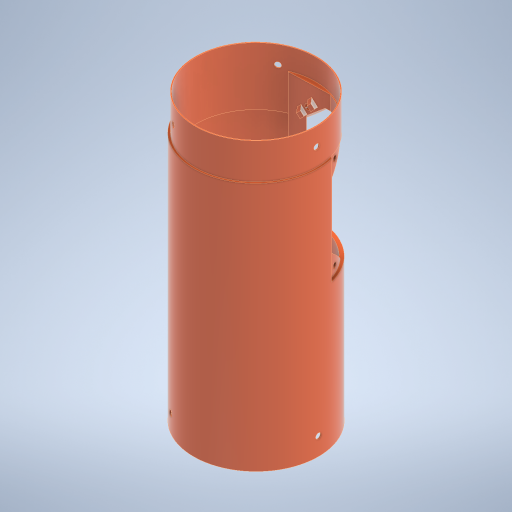
# Autodesk Inventor part: Lower skin
Saved by Autodesk Inventor 2024 (Build 280153000, 153)
## iProperties
Created: 2023-12-30
Part Number: Lower skin
Material: Plastic, Opaque White
Document SubType Name: Modeling
Designer: Jamie
Density: 0.952 g/cm^3
Appearance: Smooth - Light Orange
Author: Jamie
Autodesk Inventor part; units mm, degrees
ref_plane "XY Plane" through (0, 0, 0) normal (0, 0, 1) x (1, 0, 0)
sketch "Sketch1" plane through (0, 0, 0) normal (0, 1, 0) x (-1, 0, 0)
  circle A0 centre (0, 0) radius 35
  circle A1 centre (0, 0) radius 34.5
  dimension "d0" = 70
  dimension "d1" = 69
  constraints: 2 centre point, 2 coincident
  measures "d0" diameter of A0
  measures "d1" diameter of A1
extrude "Extrusion1" add sketch "Sketch1" along normal blind 140
ref_plane "Work Plane2" through (35, 0, 0) normal (1, 0, 0) x (0, 1, 0)
sketch "Sketch4" plane through (35, 0, 0) normal (1, 0, 0) x (0, 1, 0)
  line L0 (140, -35) -> (140, 35) projected
  point P0 (0, 0)
  point P1 (10, 0)
  dimension "d48" = 10
  measures "d48" distance of point (0, 0) point (10, 0)
hole "Hole2" at (35, 10, 0) direction (-1, 0, 0) diameter 3 depth 8 tip angle 118
sketch "Sketch5" plane through (0, 140, 0) normal (0, 1, 0) x (1, 0, 0)
  circle A0 centre (0, 0) radius 34
  circle A1 centre (0, 0) radius 33.5
  dimension "d44" = 68
  dimension "d45" = 67
  constraints: 2 centre point, 2 coincident
  measures "d44" diameter of A0
  measures "d45" diameter of A1
extrude "Extrusion3" add sketch "Sketch5" along normal blind 20
sketch "Sketch6" plane through (0, 140, 0) normal (0, -1, 0) x (1, 0, 0)
  circle A0 centre (0, 0) radius 33.5
  circle A1 centre (0, 0) radius 34.5 projected
  circle A2 centre (0, 0) radius 35
  constraints: 2 centre point, 2 coincident
extrude "Extrusion4" add sketch "Sketch6" along normal blind 12.5 contours A1
ref_plane "Work Plane4" through (34, 0, 0) normal (1, 0, 0) x (0, 1, 0)
sketch "Sketch8" plane through (34, 0, 0) normal (1, 0, 0) x (0, 1, 0)
  line L0 (160, -34) -> (160, 34) projected
  line L1 (150, 0) -> (50.9315, 0)
  line L2 (140, -35) -> (140, 35) projected
  line L3 (130, 15) -> (85, 15)
  line L4 (85, 15) -> (85, -15)
  line L5 (85, -15) -> (130, -15)
  line L6 (130, -15) -> (130, 15)
  point P0 (0, 0)
  point P1 (109.4746, 0)
  dimension "d61" = 10
  dimension "d74" = 15
  dimension "d75" = 10
  dimension "d76" = 15
  dimension "d77" = 55
  constraints: 10 end point, 3 horizontal, 2 parallel, 1 perpendicular
  measures "d61" distance from line of L0 L1.start
  measures "d74" distance from line of L1 L3.start
  measures "d75" distance from line of L2 L3.start
  measures "d76" distance from line of L1 L4.end
  measures "d77" distance from line of L2 L4.end
hole "Hole4" at (34, 150, 0) direction (-1, 0, 0) diameter 3 depth 8 tip angle 118
pattern_circular "Circular Pattern2" count 3 over 360 about axis through (0, 0, 0) along (0, 1, 0) of "Hole2", "Hole4"
sketch "Sketch27" plane through (0, 160, 0) normal (0, 1, 0) x (1, 0, 0)
  circle A0 centre (0, 0) radius 33.5 projected
  line L0 (-15.7198, 29.5827) -> (33.4973, -0.4287) construction
  line L1 (8.8889, 14.5769) -> (24.1701, 39.6371) construction
  circle A1 centre (0, 0) radius 35 construction
  point P0 (18.2219, 29.8825)
  dimension "d174" = 57.6455
  dimension "d175" = 28.823
  dimension "d176" = 0
  constraints: 4 end point, 2 point on circle, 1 perpendicular, 1 point on line, 2 other
  measures "d174" distance of L0.start L0.end
  measures "d175" distance of L0.start L1.start
  measures "d176" distance from line of L1 point (18.222, 29.882)
ref_plane "Work Plane12" through (18.2219, 160, -29.8825) normal (0.5206264, 0, -0.8537846) x (0, 1, 0)
sketch "Sketch28" plane through (18.2219, 160, -29.8825) normal (0.5206264, 0, -0.8537846) x (0, 1, 0)
  line L0 (-20, -35) -> (-20, 35) projected
  line L1 (-17.8725, 0) -> (-86.782, 0) construction
  line L2 (-20, 30) -> (-80, 30)
  line L3 (-80, 30) -> (-80, -30)
  line L4 (-80, -30) -> (-20, -30)
  line L5 (-20, -30) -> (-20, 30)
  point P0 (-160, 0)
  point P1 (-20, -30)
  dimension "d177" = 0
  dimension "d178" = 60
  dimension "d179" = 30
  dimension "d180" = 30
  constraints: 10 end point, 3 horizontal, 2 parallel, 1 perpendicular
  measures "d177" distance from line of L0 L2.start
  measures "d178" distance from line of L0 L3.end
  measures "d179" distance from line of L2.start L1
  measures "d180" distance from line of L3.end L1
extrude "Extrusion8" cut sketch "Sketch28" against normal blind 10
ref_plane "Work Plane18" through (0, 140, 0) normal (0, 1, 0) x (1, 0, 0)
ref_plane "Work Plane20" through (0, 80, 0) normal (0, 1, 0) x (1, 0, 0)
ref_plane "Work Plane23" through (25.5107, 0, -41.8354) normal (-0.8537846, 0, -0.5206264) x (0, 1, 0)
ref_plane "Work Plane21" through (-7.8977, 0, -34.0973) normal (-0.2256487, 0, -0.9742087) x (0, -1, 0)
ref_plane "Work Plane22" through (33.929, 0, -8.5919) normal (0.9694008, 0, -0.2454835) x (0, 1, 0)
ref_plane "Work Plane30" through (0, 110, 0) normal (0, 1, 0) x (1, 0, 0)
sketch "Sketch58" plane through (0, 127.5, 0) normal (0, -1, 0) x (1, 0, 0)
  line L0 (0, 0) -> (-6.1673, -33.7438) construction
  arc A0 (-6.023, -32.9541) -> (32.0543, -9.7351) centre (0, 0) ccw construction
  line L1 (0, 0) -> (32.9079, -9.9944) construction
  line L2 (0, 0) -> (33.3779, -2.8579) construction
  circle A1 centre (0, 0) radius 33.5 construction
  line L3 (0, 0) -> (-12.7429, -30.9817) construction
  arc A2 (32.0543, -9.7351) -> (33.3779, -2.8579) centre (0, 0) ccw
  arc A3 (-12.7429, -30.9817) -> (-6.023, -32.9541) centre (0, 0) ccw
  line L4 (33.3779, -2.8579) -> (34.3742, -2.9432)
  circle A4 centre (0, 0) radius 34.5 projected
  line L5 (-12.7429, -30.9817) -> (-13.1233, -31.9066)
  line L6 (32.0543, -9.7351) -> (33.3094, -8.9698)
  line L7 (33.929, -8.5919) -> (32.6898, -9.3476) projected
  line L8 (-7.2831, -33.7225) -> (-6.023, -32.9541) projected
  line L9 (-7.2831, -33.7225) -> (-6.023, -32.9541)
  point P0 (9.3407, -32.1714)
  point P1 (24.3235, -23.0351)
  point P2 (-7.228, -33.6889)
  point P3 (33.3144, -8.9667)
  dimension "d496" = 12
  dimension "d498" = 12
  dimension "d501" = 33.5
  dimension "d504" = 0
  constraints: 16 end point, 7 point on circle, 2 centre point, 2 line through centre, 2 point on line, 1 coincident, 1 collinear, 1 midpoint
  measures "d496" angle of L2 L1
  measures "d498" angle of L3 L0
  measures "d501" radius of A2
  measures "d504" distance of A3.end L8.end
extrude "Extrusion19" add sketch "Sketch58" along normal blind 47.5 contours A2 L4 A4 L7 L6 | L5 A3 L8 A4
sketch "Sketch59" plane through (0, 80, 0) normal (0, -1, 0) x (1, 0, 0)
  arc A0 (33.3779, -2.8579) -> (-12.7429, -30.9817) centre (0, 0) ccw projected
  line L0 (33.3779, -2.8579) -> (34.3742, -2.9432) projected
  arc A1 (-12.7429, -30.9817) -> (33.3779, -2.8579) centre (0, 0) ccw
  line L1 (33.3779, -2.8579) -> (34.3742, -2.9432)
  line L2 (-12.7429, -30.9817) -> (-13.1211, -31.9075)
  circle A2 centre (0, 0) radius 34.5 projected
  line L3 (-12.7429, -30.9817) -> (-13.1233, -31.9066) projected
  point P0 (32.0543, -9.7351)
  point P1 (-6.023, -32.9541)
  constraints: 4 end point, 3 point on circle, 1 centre point, 1 coincident, 1 collinear, 1 line through centre
extrude "Extrusion20" add sketch "Sketch59" along normal blind 8 contours L0 A2 L2 A1
sketch "Sketch60" plane through (0, 72, 0) normal (0, -1, 0) x (1, 0, 0)
  arc A0 (-12.7429, -30.9817) -> (33.3779, -2.8579) centre (0, 0) ccw projected
  arc A1 (-12.7429, -30.9817) -> (33.3779, -2.8579) centre (0, 0) ccw
  line L0 (-13.1211, -31.9075) -> (-12.7429, -30.9817)
  line L1 (33.3779, -2.8579) -> (34.3742, -2.9432)
  arc A2 (-12.5527, -30.5193) -> (32.8797, -2.8153) centre (0, 0) ccw
  line L2 (-12.5527, -30.5193) -> (-12.7429, -30.9817)
  line L3 (32.8797, -2.8153) -> (33.3779, -2.8579)
  circle A3 centre (0, 0) radius 34.5 projected
  line L4 (-12.5527, -30.5193) -> (10.4338, -31.3071)
  line L5 (32.8797, -2.8153) -> (23.0546, -23.6111)
  point P0 (12.4473, -30.5625)
  dimension "d505" = 33
  dimension "d519" = 23
  dimension "d520" = 23
  constraints: 12 end point, 8 point on circle, 2 centre point, 2 line through centre, 1 coincident, 1 concentric
  measures "d505" radius of A2
  measures "d519" distance of L2.start L4.end
  measures "d520" distance of L3.start L5.end
extrude "Extrusion21" add sketch "Sketch60" against normal blind 76 contours L2 A2 L3 A0 | L4 A2 | A2 L5
sketch "Sketch61" plane through (18.2219, 160, -29.8825) normal (0.5206264, 0, -0.8537846) x (0, 1, 0)
  line L0 (-80, -22.2991) -> (-20, -22.2991) projected
  line L1 (-32.5, -22.2991) -> (-67.5, -22.2991)
  line L2 (-20, 22.2991) -> (-80, 22.2991) projected
  line L3 (-32.5, 22.2991) -> (-67.5, 22.2991)
  line L4 (-32.5, 22.2991) -> (-20, 9.7991)
  line L5 (-20, -23.0434) -> (-20, 23.0434) projected
  line L6 (-20, -34) -> (-20, 34) projected
  line L7 (-20, -9.7991) -> (-32.5, -22.2991)
  line L8 (-67.5, -22.2991) -> (-80, -9.7991)
  line L9 (-80, -9.7991) -> (-80, 9.7991)
  line L10 (-80, -22.2991) -> (-80, 22.2991) projected
  line L11 (-67.5, 22.2991) -> (-80, 9.7991)
  point P0 (-160, 0)
  dimension "d508" = 45
  dimension "d509" = 45
  dimension "d510" = 45
  dimension "d511" = 45
  dimension "d512" = 12.5
  dimension "d513" = 12.5
  dimension "d514" = 12.5
  dimension "d515" = 12.5
  constraints: 14 end point, 7 point on line, 1 vertical
  measures "d508" angle of L11 L10
  measures "d509" angle of L8 L0
  measures "d510" angle of L7 L0
  measures "d511" angle of L5 L4
  measures "d512" distance of L1.start L0.end
  measures "d513" distance of L4.end L2.start
  measures "d514" distance of L2.end L9.end
  measures "d515" distance of L8.end L0.start
extrude "Extrusion22" cut sketch "Sketch61" against normal blind 10 contours L8 L9 L11 L2 L4 L5 L7 L0
sketch "Sketch62" plane through (32.8797, 72, -2.8153) normal (-0.9041677, 0, 0.4271776) x (0.4271776, 0, 0.9041677)
  line L0 (-9.9685, 59.5208) -> (-9.9685, 16.4792) projected
  line L1 (-23, 8) -> (-35.3498, 8) projected
  line L2 (-35.3498, 68) -> (-23, 68) projected
  line L3 (-6.6093, 20.5) -> (-6.6093, 8) projected
  line L4 (-6.6093, 68) -> (-6.6093, 55.5) projected
  point P0 (-11.5, -72)
  point P1 (-10.6093, 12)
  point P2 (-10.6093, 64)
  dimension "d522" = 4
  dimension "d523" = 4
  dimension "d527" = 4
  dimension "d528" = 4
  measures "d522" distance from line of L1 point (-10.609, 12)
  measures "d523" distance from line of L2 point (-10.609, 64)
  measures "d527" distance from line of L3 point (-10.609, 12)
  measures "d528" distance from line of L4 point (-10.609, 64)
hole "Hole25" at (28.3476, 84, -12.4078) at (28.3476, 136, -12.4078) direction (0.9041677, 0, -0.4271776) diameter 3.1 end through all
sketch "Sketch63" plane through (-12.5527, 72, -30.5193) normal (0.0342518, 0, 0.9994132) x (0.9994132, 0, -0.0342518)
  line L0 (23, 68) -> (35.3498, 68) projected
  line L1 (6.6093, 55.5) -> (6.6093, 68) projected
  line L2 (35.3498, 8) -> (23, 8) projected
  line L3 (6.6093, 8) -> (6.6093, 20.5) projected
  point P0 (11.5, -72)
  point P1 (10.6093, 64)
  point P2 (10.6093, 12)
  dimension "d536" = 4
  dimension "d537" = 4
  dimension "d538" = 4
  dimension "d539" = 4
  measures "d536" distance from line of point (10.609, 64) L0
  measures "d537" distance from line of L1 point (10.609, 64)
  measures "d538" distance from line of L2 point (10.609, 12)
  measures "d539" distance from line of L3 point (10.609, 12)
hole "Hole26" at (-1.9496, 136, -30.8827) at (-1.9496, 84, -30.8827) direction (-0.0342518, 0, -0.9994132) diameter 3.1 end through all
sketch "Sketch64" plane through (-12.5527, 72, -30.5193) normal (0.0342518, 0, 0.9994132) x (0.9994132, 0, -0.0342518)
  circle A0 centre (10.6093, 64) radius 2.75 construction
  circle A1 centre (10.6093, 64) radius 1.55 construction
  line L0 (10.7599, 67.668) -> (14.1471, 64.4154)
  line L1 (10.7599, 67.668) -> (12.7938, 69.7862)
  line L2 (12.7938, 69.7862) -> (16.181, 66.5336)
  line L3 (16.181, 66.5336) -> (14.1471, 64.4154)
  circle A2 centre (10.6093, 12) radius 1.55 construction
  line L4 (6.6093, 20.5) -> (9.9685, 16.4792) projected
  point P0 (11.5, -72)
  dimension "d547" = 5.5
  constraints: 8 end point, 2 parallel, 1 centre point, 1 concentric, 1 tangent
  measures "d547" diameter of A0
extrude "Extrusion23" add sketch "Sketch64" along normal blind 2
pattern_circular "Circular Pattern10" count 2 over 360 about axis through (-8.3941, 136, -218.9217) along (0.0342518, 0, 0.9994132) of "Extrusion23"
ref_plane "Work Plane31" through (0, 110, 0) normal (0, 1, 0) x (-1, 0, 0)
mirror "Mirror22" about plane through (0, 110, 0) normal (0, 1, 0) of "Extrusion23", "Circular Pattern10"
sketch "Sketch65" plane through (32.8797, 72, -2.8153) normal (-0.9041677, 0, 0.4271776) x (0.4271776, 0, 0.9041677)
  circle A0 centre (-10.6093, 64) radius 2.75 construction
  circle A1 centre (-10.6093, 64) radius 1.55 construction
  line L0 (-11.2514, 66.9231) -> (-14.9156, 64.2973)
  line L1 (-11.2514, 66.9231) -> (-12.1282, 70.5375)
  line L2 (-12.1282, 70.5375) -> (-15.7924, 67.9117)
  line L3 (-15.7924, 67.9117) -> (-14.9156, 64.2973)
  point P0 (-11.5, -72)
  dimension "d555" = 5.5
  constraints: 8 end point, 2 parallel, 1 centre point, 1 concentric, 1 tangent
  measures "d555" diameter of A0
extrude "Extrusion24" add sketch "Sketch65" along normal blind 2
pattern_circular "Circular Pattern11" count 2 over 360 about axis through (198.4662, 136, -92.7811) along (-0.9041677, 0, 0.4271776) of "Extrusion24"
mirror "Mirror23" about plane through (0, 110, 0) normal (0, 1, 0) of "Extrusion24", "Circular Pattern11"
chamfer "Chamfer25" distance 2 angle 45 1 edges at (25.1078, 141.2246, -14.5834) measured on face at (25.5599, 141.2246, -14.797)
chamfer "Chamfer26" distance 2 angle 45 1 edges at (28.5661, 133.8955, -7.2635) measured on face at (29.0182, 133.8955, -7.4771)
chamfer "Chamfer27" distance 2 angle 45 1 edges at (-0.7143, 140.7271, -28.9239) measured on face at (-0.7314, 140.7271, -29.4236)
chamfer "Chamfer28" distance 2 angle 45 1 edges at (-6.4332, 134.5255, -28.7279) measured on face at (-6.4503, 134.5255, -29.2276)
chamfer "Chamfer29" distance 2 angle 45 1 edges at (-5.757, 88.1599, -28.7511) measured on face at (-5.7741, 88.1599, -29.2508)
chamfer "Chamfer30" distance 2 angle 45 1 edges at (2.671, 82.5255, -29.0399) measured on face at (2.6538, 82.5255, -29.5396)
chamfer "Chamfer31" distance 2 angle 45 1 edges at (27.9708, 89.2246, -8.5236) measured on face at (28.4229, 89.2246, -8.7372)
chamfer "Chamfer32" distance 2 angle 45 1 edges at (24.5125, 81.8955, -15.8435) measured on face at (24.9646, 81.8955, -16.0571)
body "Solid1"
